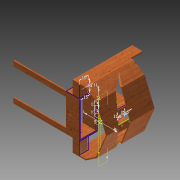
# Autodesk Inventor part: Face
Saved by Autodesk Inventor 2014 SP1 (Build 180222100, 222)
## iProperties
Created: 2017-02-19
Part Number: Face
Material: Madera (cerezo)
Document SubType Name: Modeling
Designer: Tizon
Density: 0.63 g/cm^3
Appearance: Cerezo - Natural brillo bajo
Mass: 37.2094 g
Surface Area: 490.68 cm^2
Volume: 59.0626 cm^3
Author: Tizon
Autodesk Inventor part; units mm, degrees
sketch "Boceto1" plane through (0, 0, 0) normal (0, 1, 0) x (-1, 0, 0)
  line L0 (0, 0) -> (-22, 0)
  line L1 (-22, 0) -> (-22, 62)
  line L2 (-22, 62) -> (0, 62)
  line L3 (0, 62) -> (0, 0)
  dimension "d0" = 62
  dimension "d1" = 22
  constraints: 8 end point, 2 parallel, 1 horizontal, 1 perpendicular
  measures "d0" distance of L2.end L0.start
  measures "d1" distance of L1.end L2.end
extrude "Extrusión1" add sketch "Boceto1" along normal blind 30
sketch "Boceto2" plane through (22, 0, 62) normal (1, 0, 0) x (0, 0, -1)
  line L0 (62, 0) -> (0, 0) projected
  line L1 (62, 0) -> (62, 30) projected
  line L2 (0, 30) -> (62, 30) projected
  line L3 (0, 0) -> (0, 30) projected
  line L4 (2, 28) -> (60, 28)
  line L5 (60, 28) -> (60, 2)
  line L6 (60, 2) -> (2, 2)
  line L7 (2, 2) -> (2, 28)
  dimension "d4" = 2
  dimension "d5" = 2
  dimension "d6" = 2
  dimension "d7" = 2
  constraints: 8 end point, 2 parallel, 1 horizontal, 1 perpendicular
  measures "d4" distance between parallel lines of L4 L2
  measures "d5" distance between parallel lines of L3 L7
  measures "d6" distance between parallel lines of L1 L5
  measures "d7" distance between parallel lines of L0 L6
extrude "Extrusión2" cut sketch "Boceto2" against normal blind 30 contours L4 L5 L6 L7
sketch "Boceto3" plane through (0, 0, 0) normal (0, -1, 0) x (1, 0, 0)
  line L0 (0, 0) -> (22, 0) projected
  line L1 (22, 62) -> (0, 62) projected
  line L2 (22, 62) -> (7, 62)
  line L3 (7, 62) -> (7, 31)
  circle A0 centre (7, 31) radius 1
  dimension "d10" = 15
  dimension "d11" = 31
  dimension "d12" = 2
  constraints: 4 end point, 1 centre point, 1 coincident, 1 perpendicular, 1 point on line
  measures "d10" distance of L1.start L2.end
  measures "d11" distance of L2.end L3.end
  measures "d12" diameter of A0
extrude "Extrusión3" cut sketch "Boceto3" against normal blind 15
sketch "Boceto4" plane through (0, 0, 62) normal (0, 0, 1) x (1, 0, 0)
  line L0 (22, 0) -> (0, 0) projected
  line L1 (22, 0) -> (22, 30) projected
  line L2 (0, 30) -> (22, 30) projected
  line L3 (0, 0) -> (0, 30) projected
sketch "Boceto5" plane through (0, 0, 62) normal (0, 0, 1) x (1, 0, 0)
  line L0 (22, 0) -> (0, 0) projected
  line L1 (22, 0) -> (22, 30) projected
  line L2 (0, 30) -> (22, 30) projected
  line L3 (0, 0) -> (0, 30) projected
sketch "Boceto7" plane through (0, 0, 62) normal (0, 0, 1) x (1, 0, 0)
  line L0 (22, 0) -> (0, 0) projected
  line L1 (22, 0) -> (22, 30) projected
  line L2 (0, 30) -> (22, 30) projected
  line L3 (0, 0) -> (0, 30) projected
  line L4 (0, 30) -> (22, 30)
  line L5 (22, 30) -> (22, 0)
  line L6 (22, 0) -> (0, 0)
  line L7 (0, 0) -> (0, 30)
  line L8 (22, 0) -> (11, 0)
  line L9 (11, 0) -> (11, 15)
  line L10 (11, 15) -> (22, 15)
  line L11 (22, 15) -> (22, 0)
  dimension "d17" = 15
  dimension "d18" = 11
  constraints: 16 end point, 4 parallel, 2 horizontal, 2 perpendicular
  measures "d17" distance between parallel lines of L8 L10
  measures "d18" distance between parallel lines of L1 L9
sketch "Boceto9" plane through (0, 0, 62) normal (0, 0, 1) x (1, 0, 0)
  line L0 (22, 0) -> (0, 0) projected
  line L1 (22, 0) -> (22, 30) projected
  line L2 (0, 30) -> (22, 30) projected
  line L3 (0, 0) -> (0, 30) projected
sketch "Boceto10" plane through (22, 0, 62) normal (1, 0, 0) x (0, 0, -1)
  line L0 (62, 0) -> (0, 0) projected
  line L1 (0, 30) -> (62, 30) projected
  line L2 (0, 30) -> (31, 30) construction
  line L3 (31, 30) -> (31, 0) construction
  line L4 (0, 0) -> (-20, 0)
  line L5 (-20, 0) -> (-20, 15)
  line L6 (-20, 15) -> (0, 15)
  line L7 (0, 15) -> (0, 0)
  line L8 (62, 0) -> (62, 30)
  line L9 (62, 0) -> (82, 0)
  line L10 (82, 0) -> (82, 15)
  line L11 (82, 15) -> (62, 15)
  line L12 (0, 30) -> (62, 30)
  line L13 (62, 30) -> (62, 0)
  line L14 (62, 0) -> (0, 0)
  line L15 (0, 0) -> (0, 30)
  line L16 (2, 28) -> (60, 28)
  line L17 (60, 28) -> (60, 2)
  line L18 (60, 2) -> (2, 2)
  line L19 (2, 2) -> (2, 28)
  dimension "d20" = 31
  dimension "d21" = 20
  dimension "d22" = 15
  constraints: 36 end point, 6 parallel, 3 horizontal, 3 perpendicular, 3 symmetric about line, 2 midpoint
  measures "d20" distance of L1.start L2.end
  measures "d21" distance of L5.end L6.end
  measures "d22" distance of L4.end L5.end
extrude "Extrusión4" add sketch "Boceto10" against normal blind 11 contours L4 L5 L6 L7
ref_plane "Plano de trabajo3" through (0, 30, 31) normal (0, 0, 1) x (1, 0, 0)
mirror "Simetría1" about plane through (0, 30, 31) normal (0, 0, 1) of "Extrusión4"
sketch "Boceto11" plane through (0, 0, 0) normal (0, -1, 0) x (1, 0, 0)
  line L0 (11, 0) -> (11, -20) projected
  line L1 (0, 62) -> (0, 0) projected
  line L2 (11, 82) -> (33, 82)
  line L3 (33, 82) -> (33, 84)
  line L4 (33, 84) -> (11, 84)
  line L5 (11, 84) -> (11, 82)
  line L6 (0, 31) -> (103.8517, 31) construction
  line L7 (11, 62) -> (11, 0) construction
  circle A0 centre (11, 31) radius 57.3847 construction
  line L8 (33, 84) -> (51.3255, 71.8272)
  line L9 (51.3255, 71.8272) -> (68.3847, 31)
  line L10 (33, 82) -> (50.3824, 70.4536)
  line L11 (50.3824, 70.4536) -> (66.8677, 31)
  line L12 (68.3847, 31) -> (66.8677, 31)
  line L13 (11, -20) -> (33, -20)
  line L14 (33, -20) -> (33, -22)
  line L15 (33, -22) -> (11, -22)
  line L16 (11, -22) -> (11, -20)
  line L17 (33, -22) -> (51.3255, -9.8272)
  line L18 (51.3255, -9.8272) -> (68.3847, 31)
  line L19 (33, -20) -> (50.3824, -8.4536)
  line L20 (50.3824, -8.4536) -> (66.8677, 31)
  dimension "d25" = 22
  dimension "d26" = 2
  dimension "d27" = 22
  dimension "d28" = 39.4536
  constraints: 38 end point, 5 symmetric about line, 4 parallel, 3 point on circle, 2 collinear, 2 midpoint, 2 perpendicular, 2 point on line, 1 centre point, 1 horizontal
  measures "d25" distance of L4.end L3.end
  measures "d26" distance of L4.end L2.start
  measures "d27" distance of L3.end L8.end
  measures "d28" vertical distance of L10.end L11.end
extrude "Extrusión5" add sketch "Boceto11" against normal blind 100
ref_plane "Plano de trabajo4" through (68.3847, 0, 31) normal (1, 0, 0) x (0, 1, 0)
sketch "Boceto12" plane through (68.3847, 0, 31) normal (1, 0, 0) x (0, 1, 0)
  point P0 (0, -31)
sketch "Boceto13" plane through (68.3847, 0, 31) normal (1, 0, 0) x (0, 1, 0)
  line L0 (0, 40.8272) -> (0, 53) projected
  line L1 (0, 40.8272) -> (100, 40.8272) projected
  line L2 (100, 53) -> (100, 40.8272) projected
  line L3 (0, 53) -> (100, 53) projected
  line L4 (0, 0) -> (0, 40.8272) projected
  line L5 (0, 0) -> (100, 0) projected
  line L6 (100, 40.8272) -> (100, 0) projected
  line L7 (0, 40.8272) -> (100, 40.8272) projected
  line L8 (0, -40.8272) -> (0, 0) projected
  line L9 (0, -40.8272) -> (100, -40.8272) projected
  line L10 (100, 0) -> (100, -40.8272) projected
  line L11 (0, 0) -> (100, 0) projected
  line L12 (0, -53) -> (0, -40.8272) projected
  line L13 (0, -53) -> (100, -53) projected
  line L14 (100, -40.8272) -> (100, -53) projected
  line L15 (0, -40.8272) -> (100, -40.8272) projected
  line L16 (0, 0) -> (20, 0) construction
  line L17 (0, -51) -> (100, -51) projected
  line L18 (20, 0) -> (32.1544, -40.8272)
  line L19 (32.1544, -40.8272) -> (53.0672, -51)
  line L20 (32.1544, -40.8272) -> (42.1544, -40.8272) construction
  line L21 (20, 0) -> (40, 0) construction
  line L22 (40, 0) -> (42.1544, -40.8272)
  line L23 (42.1544, -40.8272) -> (53.0672, -51)
  line L24 (40, 0) -> (20, 0)
  line L25 (20, 0) -> (0, 0)
  line L26 (42.1544, -40.8272) -> (32.1544, -40.8272)
  line L27 (0, 51) -> (100, 51) projected
  line L28 (20, 0) -> (32.1544, 40.8272)
  line L29 (32.1544, 40.8272) -> (53.0672, 51)
  line L30 (40, 0) -> (42.1544, 40.8272)
  line L31 (42.1544, 40.8272) -> (53.0672, 51)
  point P0 (0, -31)
  dimension "d32" = 20
  dimension "d33" = 10
  dimension "d34" = 20
  dimension "d35" = 20.9128
  constraints: 28 end point, 5 point on line, 3 symmetric about line, 2 collinear, 1 parallel
  measures "d32" distance of L8.end L16.end
  measures "d33" distance of L18.end L20.end
  measures "d34" distance of L16.end L21.end
  measures "d35" horizontal distance of L18.end L19.end
extrude "Extrusión6" cut sketch "Boceto13" against normal blind 40 contours L5 L22 L9 L18 | L9 L23 L19
ref_plane "Plano de trabajo5" through (11, 0, 31) normal (0, 0, 1) x (1, 0, 0)
mirror "Simetría2" about plane through (11, 0, 31) normal (0, 0, 1) of "Extrusión6"
sketch "Boceto14" plane through (68.3847, 0, 31) normal (1, 0, 0) x (0, 1, 0)
  line L0 (32.1544, 40.8272) -> (53.0672, 51) projected
  line L1 (53.0672, 51) -> (42.1544, 40.8272) projected
  line L2 (42.1544, 40.8272) -> (100, 40.8272) projected
  line L3 (100, 53) -> (100, 40.8272) projected
  line L4 (0, 53) -> (100, 53) projected
  line L5 (0, 40.8272) -> (0, 53) projected
  line L6 (0, 40.8272) -> (32.1544, 40.8272) projected
  line L7 (42.1544, 40.8272) -> (40, 0) projected
  line L8 (40, 0) -> (100, 0) projected
  line L9 (100, 40.8272) -> (100, 0) projected
  line L10 (42.1544, 40.8272) -> (100, 40.8272) projected
  line L11 (40, 0) -> (42.1544, -40.8272) projected
  line L12 (42.1544, -40.8272) -> (100, -40.8272) projected
  line L13 (100, 0) -> (100, -40.8272) projected
  line L14 (40, 0) -> (100, 0) projected
  line L15 (53.0672, -51) -> (32.1544, -40.8272) projected
  line L16 (0, -40.8272) -> (32.1544, -40.8272) projected
  line L17 (0, -53) -> (0, -40.8272) projected
  line L18 (0, -53) -> (100, -53) projected
  line L19 (100, -40.8272) -> (100, -53) projected
  line L20 (42.1544, -40.8272) -> (100, -40.8272) projected
  line L21 (42.1544, -40.8272) -> (53.0672, -51) projected
  line L22 (32.1544, -40.8272) -> (20, 0) projected
  line L23 (0, 0) -> (20, 0) projected
  line L24 (0, -40.8272) -> (0, 0) projected
  line L25 (0, -40.8272) -> (32.1544, -40.8272) projected
  line L26 (20, 0) -> (32.1544, 40.8272) projected
  line L27 (0, 40.8272) -> (32.1544, 40.8272) projected
  line L28 (0, 0) -> (0, 40.8272) projected
  line L29 (0, 0) -> (20, 0) projected
  line L30 (100, 53) -> (80, 53)
  line L31 (80, 53) -> (80, -53)
  line L32 (100, -53) -> (100, 53)
  line L33 (80, -53) -> (100, -53)
  point P0 (0, -31)
  dimension "d38" = 20
  constraints: 8 end point, 2 collinear, 2 point on line, 1 perpendicular
  measures "d38" distance of L3.start L30.end
extrude "Extrusión7" cut sketch "Boceto14" against normal blind 40 contours L31 L4 L3 L2 | L2 L9 L8 L31 | L8 L13 L12 L31 | L12 L19 L18 L31
sketch "Boceto15" plane through (0, 30, 0) normal (0, 1, 0) x (1, 0, 0)
  line L0 (0, 0) -> (0, -62) projected
  line L1 (22, -62) -> (22, 0) projected
  line L2 (0, -31) -> (22, -31) construction
  line L3 (22, -31) -> (22, -19.5) construction
  line L4 (22, -31) -> (22, -42.5) construction
  line L5 (0, -19.5) -> (55, -19.5)
  line L6 (55, -19.5) -> (55, -14.5)
  line L7 (55, -14.5) -> (22, -14.5)
  line L8 (22, -14.5) -> (22, -9.5)
  line L9 (22, -9.5) -> (0, -9.5)
  line L10 (0, -19.5) -> (0, -9.5)
  line L11 (0, -9.5) -> (0, -19.5)
  line L12 (0, -42.5) -> (55, -42.5)
  line L13 (55, -42.5) -> (55, -47.5)
  line L14 (55, -47.5) -> (22, -47.5)
  line L15 (22, -47.5) -> (22, -52.5)
  line L16 (22, -52.5) -> (0, -52.5)
  line L17 (0, -52.5) -> (0, -42.5)
  dimension "d41" = 11.5
  dimension "d42" = 11.5
  dimension "d43" = 55
  dimension "d44" = 5
  dimension "d45" = 5
  constraints: 32 end point, 6 perpendicular, 6 point on line, 6 symmetric about line, 2 midpoint, 1 parallel
  measures "d41" distance of L2.end L3.end
  measures "d42" distance of L2.end L4.end
  measures "d43" distance of L5.start L5.end
  measures "d44" distance of L5.end L6.end
  measures "d45" distance of L7.end L8.end
extrude "Extrusión8" add sketch "Boceto15" along normal blind 25 contours L9 L1 L5 L0 | L12 L1 L16 L0 | L1 L7 L6 L5 | L12 L13 L14 L1
ref_plane "Plano de trabajo6" through (55, 42.5, 47.5) normal (1, 0, 0) x (0, 0, -1)
sketch "Boceto16" plane through (55, 42.5, 47.5) normal (1, 0, 0) x (0, 0, -1)
  line L0 (28, -12.5) -> (33, -12.5) projected
  line L1 (33, -12.5) -> (33, 12.5) projected
  line L2 (28, 12.5) -> (33, 12.5) projected
  line L3 (28, -12.5) -> (28, 12.5) projected
  line L4 (0, -12.5) -> (5, -12.5) projected
  line L5 (5, -12.5) -> (5, 12.5) projected
  line L6 (0, 12.5) -> (5, 12.5) projected
  line L7 (0, -12.5) -> (0, 12.5) projected
  line L8 (0, -12.5) -> (10, -12.5)
  line L9 (10, -12.5) -> (10, 12.5)
  line L10 (10, 12.5) -> (0, 12.5)
  line L11 (0, 12.5) -> (0, -12.5)
  line L12 (5, 0) -> (16.5, 0) construction
  line L13 (-12.5, -40.5) -> (-12.5, -14.5) construction
  line L14 (-12.5, -14.5) -> (45.5, -14.5) construction
  line L15 (45.5, -14.5) -> (45.5, -40.5) construction
  line L16 (45.5, -40.5) -> (-12.5, -40.5) construction
  line L17 (67.5, -42.5) -> (-34.5, -42.5) construction
  line L18 (67.5, -27.5) -> (67.5, -42.5) construction
  line L19 (47.5, -27.5) -> (67.5, -27.5) construction
  line L20 (47.5, -27.5) -> (47.5, -12.5) construction
  line L21 (38, -12.5) -> (47.5, -12.5) construction
  line L22 (38, -12.5) -> (38, 12.5) construction
  line L23 (33, 12.5) -> (38, 12.5) construction
  line L24 (33, -12.5) -> (33, 12.5) construction
  line L25 (28, -12.5) -> (33, -12.5) construction
  line L26 (5, -12.5) -> (28, -12.5) construction
  line L27 (0, -12.5) -> (5, -12.5) construction
  line L28 (0, -12.5) -> (0, 12.5) construction
  line L29 (-5, 12.5) -> (0, 12.5) construction
  line L30 (-5, -12.5) -> (-5, 12.5) construction
  line L31 (-14.5, -12.5) -> (-5, -12.5) construction
  line L32 (-14.5, -27.5) -> (-14.5, -12.5) construction
  line L33 (-14.5, -27.5) -> (-34.5, -27.5) construction
  line L34 (-34.5, -27.5) -> (-34.5, -42.5) construction
  line L35 (16.5, -12.5) -> (16.5, -3.1507) construction
  line L36 (33, -12.5) -> (28, -12.5)
  line L37 (33, 12.5) -> (28, 12.5)
  line L38 (33, -12.5) -> (33, 12.5)
  line L39 (33, -12.5) -> (23, -12.5)
  line L40 (23, -12.5) -> (23, 12.5)
  line L41 (23, 12.5) -> (33, 12.5)
  point P0 (47.5, -42.5)
  dimension "d49" = 25
  dimension "d50" = 11.5
  dimension "d51" = 11.5
  constraints: 24 end point, 6 symmetric about line, 3 perpendicular, 2 midpoint, 2 parallel, 1 horizontal
  measures "d49" distance of L8.end L9.end
  measures "d50" distance of L12.start L12.end
  measures "d51" distance of L26.start L35.start
extrude "Extrusión9" add sketch "Boceto16" along normal blind 2 contours L7 L6 L5 L4 | L5 L10 L9 L8
ref_plane "Plano de trabajo7" through (33, 0, 31) normal (0, 0, -1) x (-1, 0, 0)
mirror "Simetría3" about plane through (33, 0, 31) normal (0, 0, -1) of "Extrusión9"
ref_plane "Plano de trabajo8" through (55, 42.5, 24.5) normal (-1, 0, 0) x (0, 0, 1)
sketch "Boceto17" plane through (55, 42.5, 24.5) normal (-1, 0, 0) x (0, 0, 1)
  line L0 (-5, -12.5) -> (-5, 12.5) projected
  line L1 (-5, -12.5) -> (0, -12.5) projected
  line L2 (0, -12.5) -> (0, 12.5) projected
  line L3 (0, 12.5) -> (-5, 12.5) projected
  line L4 (18, -12.5) -> (18, 12.5) projected
  line L5 (13, 12.5) -> (18, 12.5) projected
  line L6 (13, -12.5) -> (13, 12.5) projected
  line L7 (18, -12.5) -> (13, -12.5) projected
  line L8 (18, -12.5) -> (18, -5.5) construction
  line L9 (18, -5.5) -> (15.5, -5.5) construction
  circle A0 centre (15.5, -5.5) radius 1.5 construction
  circle A1 centre (15.5, -5.5) radius 1.5
  circle A2 centre (15.5, 6.5997) radius 1.5
  circle A3 centre (-2.5, 6.5997) radius 1.5
  circle A4 centre (-2.5, -5.5) radius 1.5
  point P0 (-24.5, -42.5)
  dimension "d54" = 7
  dimension "d55" = 2.5
  dimension "d56" = 3
  dimension "d57" = 3
  dimension "d58" = 3
  dimension "d59" = 3
  dimension "d60" = 3
  constraints: 5 centre point, 4 end point, 2 coincident, 1 perpendicular, 1 point on line
  measures "d54" distance of L4.start L8.end
  measures "d55" distance of L8.end L9.end
  measures "d56" diameter of A0
  measures "d57" diameter of A1
  measures "d58" diameter of A2
  measures "d59" diameter of A3
  measures "d60" diameter of A4
extrude "Extrusión10" cut sketch "Boceto17" against normal blind 5 contours A1 | A2 | A3 | A4
sketch "Boceto18" plane through (0, 0, 0) normal (0, -1, 0) x (1, 0, 0)
  line L0 (0, 62) -> (-88, 62)
  line L1 (-88, 62) -> (-88, 53.488)
  line L2 (-88, 53.488) -> (0, 53.488)
  line L3 (0, 53.488) -> (0, 62)
  dimension "d63" = 88
  constraints: 8 end point, 2 parallel, 1 horizontal, 1 perpendicular
  measures "d63" distance of L2.end L1.end
extrude "Extrusión11" add sketch "Boceto18" against normal blind 2
mirror "Simetría4" about plane through (33, 0, 31) normal (0, 0, -1) of "Extrusión11"
fillet "Empalme1" radius 2 1 edges at (27.5, 55, 19.5)
fillet "Empalme2" radius 2 1 edges at (27.5, 55, 42.5)
fillet "Empalme3" radius 2 1 edges at (56, 55, 37.5)
fillet "Empalme4" radius 2 1 edges at (56, 55, 24.5)
fillet "Empalme5" radius 2 1 edges at (11, 15, 72)
fillet "Empalme6" radius 2 1 edges at (11, 15, -10)
fillet "Empalme7" radius 2 1 edges at (22, 15, 72)
fillet "Empalme8" radius 2 1 edges at (22, 15, -10)
